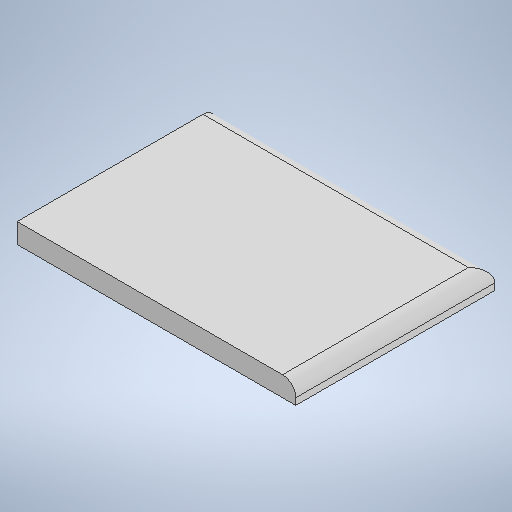
# Autodesk Inventor part: Pieza Sensor Ultrasonico
Saved by Autodesk Inventor 2025.3 (Build 293356030, 356C)
## iProperties
Created: 2026-07-17
Part Number: Pieza Sensor Ultrasonico
Material: Generic
Document SubType Name: Modeling
Designer: Samuel Correa Vega
Density: 1 g/cm^3
Appearance: Default
Author: Samuel Correa Vega
Autodesk Inventor part; units mm, degrees
note: some values were not read from the file. Chosen so that the rebuilt part matches the saved one: edges of "Fillet1".
ref_plane "YZ Plane" through (0, 0, 0) normal (1, 0, 0) x (0, 1, 0)
ref_plane "XZ Plane" through (0, 0, 0) normal (0, 1, 0) x (-1, 0, 0)
ref_plane "XY Plane" through (0, 0, 0) normal (0, 0, 1) x (1, 0, 0)
sketch "Sketch1" plane through (0, 0, 0) normal (0, 1, 0) x (-1, 0, 0)
  line L0 (21, -15) -> (-21, -15)
  line L1 (-21, -15) -> (-21, 15)
  line L2 (-21, 15) -> (21, 15)
  line L3 (21, 15) -> (21, -15)
  point P0 (0, 0)
  point P1 (0, 0)
  point P2 (-21, 0)
  point P3 (21, 0)
  point P4 (0, -15)
  dimension "d0" = 42
  dimension "d1" = 30
  constraints: 8 end point, 3 midpoint, 2 coincident, 2 horizontal alignment, 2 parallel, 1 horizontal, 1 perpendicular, 1 vertical, 1 vertical alignment
  measures "d0" distance of L0.start L0.end
  measures "d1" distance of L0.end L1.end
extrude "Extrusion1" add sketch "Sketch1" along normal blind 3
fillet "Fillet1" radius 2 2 edges at (0, 3, -15) (21, 3, 0)
body "Solid1"
